Autodesk Fusion 360 part; units mm, degrees
(part 5 of 25)
  line L540 (19.5072, 53.213) -> (18.3388, 53.213)
  arc A1749 (22.1742, 53.7803) -> (22.1742, 53.8311) centre (22.1742, 53.8057) ccw
  arc A1750 (14.1676, 51.9684) -> (14.1676, 52.0192) centre (14.1676, 51.9938) ccw
  line L541 (22.1742, 53.6758) -> (22.1742, 53.9355)
  arc A1751 (18.3388, 53.8875) -> (18.3388, 53.8367) centre (18.3388, 53.8621) ccw
  arc A1752 (14.4272, 54.983) -> (14.4272, 55.0338) centre (14.4272, 55.0084) ccw
  arc A1753 (13.2334, 52.2534) -> (13.2842, 52.2534) centre (13.2588, 52.2534) ccw
  arc A1754 (19.5326, 54.7567) -> (19.4818, 54.7567) centre (19.5072, 54.7567) ccw
  arc A1755 (7.0605, 47.7158) -> (7.019, 47.6866) centre (7.0398, 47.7012) ccw
  arc A1756 (18.3388, 53.2384) -> (18.3388, 53.1876) centre (18.3388, 53.213) ccw
  arc A1757 (18.3265, 53.2352) -> (18.3511, 53.1908) centre (18.3388, 53.213) ccw
  arc A1758 (19.4818, 54.7567) -> (19.5326, 54.7567) centre (19.5072, 54.7567) ccw
  arc A1759 (18.3134, 54.7567) -> (18.3642, 54.7567) centre (18.3388, 54.7567) ccw
  arc A1760 (13.2588, 55.0338) -> (13.2588, 54.983) centre (13.2588, 55.0084) ccw
  line L542 (18.6634, 55.0813) -> (19.1826, 55.0813)
  arc A1761 (14.4526, 52.5131) -> (14.4018, 52.5131) centre (14.4272, 52.5131) ccw
  arc A1762 (13.2457, 53.0208) -> (13.2719, 52.9772) centre (13.2588, 52.999) ccw
  arc A1763 (19.5072, 53.1876) -> (19.5072, 53.2384) centre (19.5072, 53.213) ccw
  arc A1764 (7.4038, 46.5328) -> (7.4546, 46.5328) centre (7.4292, 46.5328) ccw
  arc A1765 (18.3642, 54.7567) -> (18.3134, 54.7567) centre (18.3388, 54.7567) ccw
  arc A1766 (18.3134, 54.4322) -> (18.3642, 54.4322) centre (18.3388, 54.4322) ccw
  arc A1767 (18.6634, 55.1067) -> (18.6634, 55.0559) centre (18.6634, 55.0813) ccw
  arc A1768 (18.6634, 55.0813) -> (18.3388, 54.7567) centre (18.6634, 54.7567) ccw
  line L543 (21.0058, 54.4336) -> (22.1742, 55.0827)
  arc A1769 (11.8618, 52.2534) -> (11.9126, 52.2534) centre (11.8872, 52.2534) ccw
  arc A1770 (19.5072, 53.8367) -> (19.5072, 53.8875) centre (19.5072, 53.8621) ccw
  line L544 (14.1676, 51.9938) -> (13.5184, 51.9938)
  arc A1771 (6.3103, 47.6932) -> (6.2621, 47.7092) centre (6.2862, 47.7012) ccw
  arc A1772 (13.2842, 52.5131) -> (13.2334, 52.5131) centre (13.2588, 52.5131) ccw
  arc A1773 (13.2588, 53.8033) -> (13.2588, 53.7525) centre (13.2588, 53.7779) ccw
  line L545 (18.3388, 53.213) -> (19.5072, 53.8621)
  arc A1774 (13.5184, 52.0192) -> (13.5184, 51.9684) centre (13.5184, 51.9938) ccw
  line L546 (11.8872, 52.5131) -> (11.8872, 52.2534)
  arc A1775 (19.5072, 54.4068) -> (19.5072, 54.4576) centre (19.5072, 54.4322) ccw
  arc A1776 (14.4018, 52.2534) -> (14.4526, 52.2534) centre (14.4272, 52.2534) ccw
  arc A1777 (14.1676, 51.9938) -> (14.4272, 52.2534) centre (14.1676, 52.2534) ccw
  line L547 (13.2588, 52.999) -> (13.9079, 53.3885)
  arc A1778 (14.4272, 54.3339) -> (14.4272, 54.3847) centre (14.4272, 54.3593) ccw
  line L548 (19.5072, 53.8621) -> (18.3388, 53.8621)
  arc A1779 (22.1822, 52.8672) -> (22.1662, 52.9154) centre (22.1742, 52.8913) ccw
  line L549 (19.5072, 54.7567) -> (19.5072, 54.4322)
  arc A1780 (22.1662, 52.8672) -> (22.1822, 52.9154) centre (22.1742, 52.8913) ccw
  arc A1781 (18.3388, 52.2534) -> (18.5984, 51.9938) centre (18.5984, 52.2534) ccw
  line L550 (14.4272, 52.999) -> (13.2588, 52.999)
  arc A1782 (13.921, 53.3667) -> (13.8948, 53.4103) centre (13.9079, 53.3885) ccw
  arc A1783 (19.5195, 53.8399) -> (19.4949, 53.8843) centre (19.5072, 53.8621) ccw
  arc A1784 (19.5072, 54.7567) -> (19.1826, 55.0813) centre (19.1826, 54.7567) ccw
  arc A1785 (19.1826, 55.1067) -> (19.1826, 55.0559) centre (19.1826, 55.0813) ccw
  arc A1786 (13.2588, 53.0244) -> (13.2588, 52.9736) centre (13.2588, 52.999) ccw
  line L551 (13.2588, 53.7779) -> (14.4272, 53.7779)
  arc A1787 (14.4272, 53.7525) -> (14.4272, 53.8033) centre (14.4272, 53.7779) ccw
  arc A1788 (18.6634, 55.0559) -> (18.6634, 55.1067) centre (18.6634, 55.0813) ccw
  line L552 (18.3388, 54.4322) -> (18.3388, 54.7567)
  arc A1789 (18.3388, 54.4576) -> (18.3388, 54.4068) centre (18.3388, 54.4322) ccw
  arc A1790 (6.6516, 46.5248) -> (6.6998, 46.5408) centre (6.6757, 46.5328) ccw
  arc A1791 (19.4818, 54.4322) -> (19.5326, 54.4322) centre (19.5072, 54.4322) ccw
  arc A1792 (19.1826, 55.0559) -> (19.1826, 55.1067) centre (19.1826, 55.0813) ccw
  arc A1793 (14.4526, 52.2534) -> (14.4018, 52.2534) centre (14.4272, 52.2534) ccw
  arc A1794 (13.5184, 51.9684) -> (13.5184, 52.0192) centre (13.5184, 51.9938) ccw
  line L553 (13.2588, 52.2534) -> (13.2588, 52.5131)
  arc A1795 (13.2588, 52.2534) -> (13.5184, 51.9938) centre (13.5184, 52.2534) ccw
  arc A1796 (13.2842, 52.2534) -> (13.2334, 52.2534) centre (13.2588, 52.2534) ccw
  line L554 (13.9079, 53.3885) -> (13.2588, 53.7779)
  line L555 (14.4272, 52.5131) -> (14.4272, 52.2534)
  arc A1797 (13.2719, 53.7997) -> (13.2457, 53.7562) centre (13.2588, 53.7779) ccw
  arc A1798 (13.8948, 53.3667) -> (13.921, 53.4103) centre (13.9079, 53.3885) ccw
  line L556 (14.4272, 54.3593) -> (13.2588, 54.3593)
  line L557 (13.2588, 54.3593) -> (14.4272, 55.0084)
  arc A1799 (16.9926, 53.5987) -> (16.9418, 53.5987) centre (16.9672, 53.5987) ccw
  arc A1800 (16.7076, 51.9938) -> (16.9672, 52.2534) centre (16.7076, 52.2534) ccw
  line L558 (16.9672, 52.9496) -> (16.9672, 53.5987)
  arc A1801 (11.9126, 52.2534) -> (11.8618, 52.2534) centre (11.8872, 52.2534) ccw
  arc A1802 (15.8242, 52.2534) -> (15.7734, 52.2534) centre (15.7988, 52.2534) ccw
  arc A1803 (14.1676, 52.0192) -> (14.1676, 51.9684) centre (14.1676, 51.9938) ccw
  line L559 (11.8872, 52.9496) -> (11.8872, 53.5987)
  arc A1804 (10.6934, 52.2534) -> (10.7442, 52.2534) centre (10.7188, 52.2534) ccw
  arc A1805 (63.6552, 12.3105) -> (63.6044, 12.3105) centre (63.6298, 12.3105) ccw
  arc A1806 (16.9672, 53.2488) -> (16.9672, 53.2996) centre (16.9672, 53.2742) ccw
  arc A1807 (11.8707, 52.9303) -> (11.9037, 52.969) centre (11.8872, 52.9497) ccw
  line L560 (15.7988, 52.2534) -> (15.7988, 52.5131)
  line L561 (16.9672, 52.5131) -> (16.9672, 52.2534)
  line L562 (16.0584, 52.9496) -> (15.7988, 53.2742)
  arc A1808 (10.7188, 52.2534) -> (10.9784, 51.9938) centre (10.9784, 52.2534) ccw
  arc A1809 (10.9706, 52.9255) -> (10.9863, 52.9738) centre (10.9784, 52.9497) ccw
  line L563 (11.2381, 53.5014) -> (11.8872, 52.9496)
  arc A1810 (14.4272, 52.9736) -> (14.4272, 53.0244) centre (14.4272, 52.999) ccw
  line L564 (14.4272, 55.0084) -> (13.2588, 55.0084)
  arc A1811 (13.2588, 54.3847) -> (13.2588, 54.3339) centre (13.2588, 54.3593) ccw
  arc A1812 (16.9418, 52.9496) -> (16.9926, 52.9496) centre (16.9672, 52.9496) ccw
  arc A1813 (10.7442, 52.5131) -> (10.6934, 52.5131) centre (10.7188, 52.5131) ccw
  arc A1814 (16.9926, 52.2534) -> (16.9418, 52.2534) centre (16.9672, 52.2534) ccw
  arc A1815 (11.0109, 53.5733) -> (11.0109, 53.6241) centre (11.0109, 53.5987) ccw
  line L565 (15.7988, 53.2742) -> (16.9672, 53.2742)
  arc A1816 (13.2465, 54.3815) -> (13.2711, 54.3371) centre (13.2588, 54.3593) ccw
  arc A1817 (14.4395, 54.9862) -> (14.4149, 55.0306) centre (14.4272, 55.0084) ccw
  arc A1818 (10.7442, 53.3066) -> (10.6934, 53.3066) centre (10.7188, 53.3066) ccw
  arc A1819 (63.6044, 10.2362) -> (63.6552, 10.2362) centre (63.6298, 10.2362) ccw
  arc A1820 (63.6552, 9.7197) -> (63.6044, 9.7197) centre (63.6298, 9.7197) ccw
  arc A1821 (11.9126, 53.5987) -> (11.8618, 53.5987) centre (11.8872, 53.5987) ccw
  arc A1822 (11.6276, 51.9684) -> (11.6276, 52.0192) centre (11.6276, 51.9938) ccw
  arc A1823 (10.9784, 52.0192) -> (10.9784, 51.9684) centre (10.9784, 51.9938) ccw
  arc A1824 (11.2545, 53.5207) -> (11.2216, 53.482) centre (11.2381, 53.5014) ccw
  arc A1825 (16.0584, 52.0192) -> (16.0584, 51.9684) centre (16.0584, 51.9938) ccw
  arc A1826 (63.6552, 11.0151) -> (63.6044, 11.0151) centre (63.6298, 11.0151) ccw
  arc A1827 (16.7076, 52.0192) -> (16.7076, 51.9684) centre (16.7076, 51.9938) ccw
  arc A1828 (10.6934, 53.3066) -> (10.7442, 53.3066) centre (10.7188, 53.3066) ccw
  arc A1829 (15.7988, 52.2534) -> (16.0584, 51.9938) centre (16.0584, 52.2534) ccw
  arc A1830 (16.0386, 52.9338) -> (16.0783, 52.9655) centre (16.0585, 52.9497) ccw
  arc A1831 (16.9418, 52.2534) -> (16.9926, 52.2534) centre (16.9672, 52.2534) ccw
  line L566 (16.7076, 51.9938) -> (16.0584, 51.9938)
  line L567 (63.6298, 10.2362) -> (63.6298, 11.0151)
  arc A1832 (11.0109, 53.6241) -> (11.0109, 53.5733) centre (11.0109, 53.5987) ccw
  line L568 (19.5072, 54.4322) -> (18.3388, 54.4322)
  arc A1833 (15.8242, 52.5131) -> (15.7734, 52.5131) centre (15.7988, 52.5131) ccw
  arc A1834 (11.2197, 53.4838) -> (11.2565, 53.5189) centre (11.2381, 53.5014) ccw
  arc A1835 (15.7988, 53.2996) -> (15.7988, 53.2488) centre (15.7988, 53.2742) ccw
  arc A1836 (10.7188, 53.3066) -> (10.9784, 52.9496) centre (11.094, 53.3066) ccw
  arc A1837 (16.0584, 51.9684) -> (16.0584, 52.0192) centre (16.0584, 51.9938) ccw
  arc A1838 (16.7076, 51.9684) -> (16.7076, 52.0192) centre (16.7076, 51.9938) ccw
  line L569 (63.6298, 8.9408) -> (63.6298, 9.7197)
  arc A1839 (10.7442, 52.2534) -> (10.6934, 52.2534) centre (10.7188, 52.2534) ccw
  line L570 (11.6276, 51.9938) -> (10.9784, 51.9938)
  arc A1840 (15.7734, 52.2534) -> (15.8242, 52.2534) centre (15.7988, 52.2534) ccw
  arc A1841 (11.6276, 51.9938) -> (11.8872, 52.2534) centre (11.6276, 52.2534) ccw
  line L571 (63.6298, 11.5316) -> (63.6298, 12.3105)
  arc A1842 (11.0109, 53.5987) -> (10.7188, 53.3066) centre (11.0109, 53.3066) ccw
  arc A1843 (11.8618, 52.9496) -> (11.9126, 52.9496) centre (11.8872, 52.9496) ccw
  arc A1844 (63.6044, 11.5316) -> (63.6552, 11.5316) centre (63.6298, 11.5316) ccw
  arc A1845 (63.6044, 8.9408) -> (63.6552, 8.9408) centre (63.6298, 8.9408) ccw
  line L572 (63.6298, 12.827) -> (63.6298, 13.6059)
  line L573 (68.7098, 8.9408) -> (68.7098, 9.7197)
  arc A1846 (15.8186, 53.29) -> (15.779, 53.2583) centre (15.7988, 53.2742) ccw
  arc A1847 (45.9813, 26.1699) -> (46.0259, 26.1456) centre (46.0036, 26.1577) ccw
  line L574 (45.5168, 27.1408) -> (45.5168, 27.66)
  line L575 (68.7098, 12.827) -> (68.7098, 13.6059)
  arc A1848 (10.9784, 51.9684) -> (10.9784, 52.0192) centre (10.9784, 51.9938) ccw
  line L576 (66.1698, 12.827) -> (66.1698, 13.6059)
  arc A1849 (11.2381, 53.5014) -> (11.0109, 53.5987) centre (11.011, 53.285) ccw
  arc A1850 (45.5422, 26.2876) -> (45.4914, 26.2876) centre (45.5168, 26.2876) ccw
  arc A1851 (45.5168, 27.1662) -> (45.5168, 27.1154) centre (45.5168, 27.1408) ccw
  arc A1852 (46.6852, 27.1154) -> (46.6852, 27.1662) centre (46.6852, 27.1408) ccw
  arc A1853 (46.5229, 25.9955) -> (46.6852, 26.385) centre (46.1367, 26.385) ccw
  arc A1854 (46.505, 26.0135) -> (46.5408, 25.9775) centre (46.5229, 25.9955) ccw
  arc A1855 (46.6598, 26.385) -> (46.7106, 26.385) centre (46.6852, 26.385) ccw
  arc A1856 (46.1765, 26.5277) -> (46.2203, 26.5019) centre (46.1984, 26.5148) ccw
  line L577 (10.7188, 52.2534) -> (10.7188, 52.5131)
  arc A1857 (66.1952, 12.3105) -> (66.1444, 12.3105) centre (66.1698, 12.3105) ccw
  arc A1858 (66.1952, 9.7197) -> (66.1444, 9.7197) centre (66.1698, 9.7197) ccw
  arc A1859 (66.1952, 13.6059) -> (66.1444, 13.6059) centre (66.1698, 13.6059) ccw
  arc A1860 (46.4256, 26.6192) -> (46.4256, 26.67) centre (46.4256, 26.6446) ccw
  line L578 (68.7098, 11.5316) -> (68.7098, 12.3105)
  arc A1861 (68.6844, 11.5316) -> (68.7352, 11.5316) centre (68.7098, 11.5316) ccw
  arc A1862 (45.7764, 26.028) -> (46.0036, 26.1578) centre (45.7764, 26.2917) ccw
  arc A1863 (45.6345, 26.5645) -> (45.5938, 26.5949) centre (45.6142, 26.5797) ccw
  arc A1864 (68.6844, 10.2362) -> (68.7352, 10.2362) centre (68.7098, 10.2362) ccw
  line L579 (63.6298, 14.1224) -> (63.6298, 14.9013)
  line L580 (68.7098, 10.2362) -> (68.7098, 11.0151)
  arc A1865 (66.1952, 11.0151) -> (66.1444, 11.0151) centre (66.1698, 11.0151) ccw
  arc A1866 (68.7352, 13.6059) -> (68.6844, 13.6059) centre (68.7098, 13.6059) ccw
  arc A1867 (66.1444, 14.1224) -> (66.1952, 14.1224) centre (66.1698, 14.1224) ccw
  arc A1868 (68.6844, 12.827) -> (68.7352, 12.827) centre (68.7098, 12.827) ccw
  arc A1869 (68.7352, 9.7197) -> (68.6844, 9.7197) centre (68.7098, 9.7197) ccw
  arc A1870 (63.6044, 14.1224) -> (63.6552, 14.1224) centre (63.6298, 14.1224) ccw
  line L581 (66.1698, 10.2362) -> (66.1698, 11.0151)
  arc A1871 (45.5422, 27.66) -> (45.4914, 27.66) centre (45.5168, 27.66) ccw
  line L582 (46.1984, 26.5148) -> (46.0036, 26.1578)
  arc A1872 (66.1444, 11.5316) -> (66.1952, 11.5316) centre (66.1698, 11.5316) ccw
  arc A1873 (46.7106, 26.385) -> (46.6598, 26.385) centre (46.6852, 26.385) ccw
  line L583 (66.1698, 11.5316) -> (66.1698, 12.3105)
  arc A1874 (46.6852, 26.385) -> (46.4256, 26.6446) centre (46.4256, 26.385) ccw
  arc A1875 (68.7352, 11.0151) -> (68.6844, 11.0151) centre (68.7098, 11.0151) ccw
  arc A1876 (68.7352, 12.3105) -> (68.6844, 12.3105) centre (68.7098, 12.3105) ccw
  line L584 (66.1698, 8.9408) -> (66.1698, 9.7197)
  arc A1877 (68.7352, 14.9013) -> (68.6844, 14.9013) centre (68.7098, 14.9013) ccw
  arc A1878 (45.6142, 26.5797) -> (45.5168, 26.2876) centre (46.0036, 26.2876) ccw
  arc A1879 (66.1952, 14.9013) -> (66.1444, 14.9013) centre (66.1698, 14.9013) ccw
  arc A1880 (45.7764, 26.0533) -> (45.7764, 26.0026) centre (45.7764, 26.028) ccw
  arc A1881 (63.6552, 13.6059) -> (63.6044, 13.6059) centre (63.6298, 13.6059) ccw
  arc A1882 (16.9926, 52.5131) -> (16.9418, 52.5131) centre (16.9672, 52.5131) ccw
  arc A1883 (11.9126, 52.5131) -> (11.8618, 52.5131) centre (11.8872, 52.5131) ccw
  arc A1884 (63.6552, 14.9013) -> (63.6044, 14.9013) centre (63.6298, 14.9013) ccw
  line L585 (46.6852, 27.1408) -> (45.5168, 27.1408)
  line L586 (68.7098, 14.1224) -> (68.7098, 14.9013)
  arc A1885 (46.7106, 27.66) -> (46.6598, 27.66) centre (46.6852, 27.66) ccw
  arc A1886 (45.4914, 26.2876) -> (45.5422, 26.2876) centre (45.5168, 26.2876) ccw
  arc A1887 (66.1444, 10.2362) -> (66.1952, 10.2362) centre (66.1698, 10.2362) ccw
  arc A1888 (11.6276, 52.0192) -> (11.6276, 51.9684) centre (11.6276, 51.9938) ccw
  arc A1889 (46.4256, 26.67) -> (46.4256, 26.6192) centre (46.4256, 26.6446) ccw
  arc A1890 (45.4914, 27.1408) -> (45.5422, 27.1408) centre (45.5168, 27.1408) ccw
  arc A1891 (63.6044, 12.827) -> (63.6552, 12.827) centre (63.6298, 12.827) ccw
  line L587 (46.0361, 27.1408) -> (46.0361, 27.5302)
  line L588 (66.1698, 14.1224) -> (66.1698, 14.9013)
  arc A1892 (66.1444, 12.827) -> (66.1952, 12.827) centre (66.1698, 12.827) ccw
  arc A1893 (46.2207, 26.5026) -> (46.1761, 26.5269) centre (46.1984, 26.5148) ccw
  line L589 (46.6852, 27.66) -> (46.6852, 27.1408)
  line L590 (48.5902, 28.091) -> (47.4218, 28.091)
  arc A1894 (45.8414, 30.4405) -> (45.8414, 30.3897) centre (45.8414, 30.4151) ccw
  arc A1895 (47.4416, 29.6125) -> (47.402, 29.5808) centre (47.4218, 29.5966) ccw
  arc A1896 (46.0107, 27.1408) -> (46.0615, 27.1408) centre (46.0361, 27.1408) ccw
  arc A1897 (45.4914, 28.461) -> (45.5422, 28.461) centre (45.5168, 28.461) ccw
  arc A1898 (45.8414, 31.0896) -> (45.8414, 31.0388) centre (45.8414, 31.0642) ccw
  arc A1899 (47.4472, 28.4155) -> (47.3964, 28.4155) centre (47.4218, 28.4155) ccw
  arc A1900 (46.3606, 30.3897) -> (46.3606, 30.4405) centre (46.3606, 30.4151) ccw
  line L591 (47.7464, 28.7401) -> (48.2656, 28.7401)
  arc A1901 (47.4218, 29.622) -> (47.4218, 29.5712) centre (47.4218, 29.5966) ccw
  line L592 (48.5902, 29.2721) -> (48.5902, 29.9212)
  arc A1902 (45.5168, 28.1619) -> (45.5168, 28.1111) centre (45.5168, 28.1365) ccw
  arc A1903 (66.1444, 8.9408) -> (66.1952, 8.9408) centre (66.1698, 8.9408) ccw
  arc A1904 (45.5168, 26.2876) -> (45.7764, 26.028) centre (45.7764, 26.2876) ccw
  arc A1905 (46.3606, 30.4405) -> (46.3606, 30.3897) centre (46.3606, 30.4151) ccw
  line L593 (46.6852, 29.5966) -> (45.5168, 29.9861)
  arc A1906 (47.3964, 28.4155) -> (47.4472, 28.4155) centre (47.4218, 28.4155) ccw
  line L594 (48.5902, 28.4155) -> (48.5902, 28.091)
  arc A1907 (45.4914, 28.1365) -> (45.5422, 28.1365) centre (45.5168, 28.1365) ccw
  arc A1908 (46.0255, 26.1449) -> (45.9818, 26.1707) centre (46.0037, 26.1578) ccw
  arc A1909 (48.5648, 28.4156) -> (48.6156, 28.4155) centre (48.5902, 28.4155) ccw
  line L595 (46.6852, 28.1365) -> (45.5168, 28.1365)
  arc A1910 (47.7464, 28.7147) -> (47.7464, 28.7655) centre (47.7464, 28.7401) ccw
  line L596 (45.5168, 29.2072) -> (46.6852, 29.5966)
  arc A1911 (45.5248, 30.0102) -> (45.5088, 29.962) centre (45.5168, 29.9861) ccw
  arc A1912 (46.4256, 26.6446) -> (46.1984, 26.5148) centre (46.4256, 26.3809) ccw
  arc A1913 (47.7464, 28.7401) -> (47.4218, 28.4155) centre (47.7464, 28.4155) ccw
  arc A1914 (48.5902, 28.0656) -> (48.5902, 28.1164) centre (48.5902, 28.091) ccw
  arc A1915 (46.6932, 29.5726) -> (46.6772, 29.6207) centre (46.6852, 29.5967) ccw
  arc A1916 (46.1405, 28.1365) -> (46.1913, 28.1365) centre (46.1659, 28.1365) ccw
  arc A1917 (46.6598, 27.1408) -> (46.7106, 27.1408) centre (46.6852, 27.1408) ccw
  arc A1918 (46.6852, 28.1111) -> (46.6852, 28.1619) centre (46.6852, 28.1365) ccw
  line L597 (47.4218, 28.091) -> (47.4218, 28.4155)
  arc A1919 (45.5088, 29.2313) -> (45.5248, 29.1831) centre (45.5168, 29.2072) ccw
  arc A1920 (46.3606, 30.4151) -> (46.3606, 31.0642) centre (46.3606, 30.7396) ccw
  arc A1921 (48.2656, 28.7147) -> (48.2656, 28.7655) centre (48.2656, 28.7401) ccw
  line L598 (46.1659, 28.461) -> (46.1659, 28.1365)
  line L599 (45.5168, 28.1365) -> (45.5168, 28.461)
  arc A1922 (48.2656, 28.7655) -> (48.2656, 28.7147) centre (48.2656, 28.7401) ccw
  line L600 (45.8414, 31.0642) -> (46.3606, 31.0642)
  arc A1923 (48.5902, 28.4155) -> (48.2656, 28.7401) centre (48.2656, 28.4155) ccw
  arc A1924 (47.6616, 29.2562) -> (47.7013, 29.288) centre (47.6814, 29.2721) ccw
  line L601 (47.4218, 29.5966) -> (48.5902, 29.5966)
  arc A1925 (45.5422, 28.461) -> (45.4914, 28.461) centre (45.5168, 28.461) ccw
  arc A1926 (45.8414, 31.0642) -> (45.8414, 30.4151) centre (45.8414, 30.7396) ccw
  arc A1927 (68.6844, 14.1224) -> (68.7352, 14.1224) centre (68.7098, 14.1224) ccw
  arc A1928 (47.3964, 28.091) -> (47.4472, 28.091) centre (47.4218, 28.091) ccw
  arc A1929 (48.5648, 28.091) -> (48.6156, 28.091) centre (48.5902, 28.091) ccw
  arc A1930 (45.7764, 26.0025) -> (45.7764, 26.0534) centre (45.7764, 26.028) ccw
  line L602 (47.6814, 29.2721) -> (47.4218, 29.5966)
  arc A1931 (46.1659, 28.461) -> (45.5168, 28.461) centre (45.8414, 28.461) ccw
  arc A1932 (46.3606, 31.0896) -> (46.3606, 31.0388) centre (46.3606, 31.0642) ccw
  arc A1933 (45.8414, 30.3897) -> (45.8414, 30.4405) centre (45.8414, 30.4151) ccw
  arc A1934 (68.6844, 8.9408) -> (68.7352, 8.9408) centre (68.7098, 8.9408) ccw
  arc A1935 (48.5902, 29.5712) -> (48.5902, 29.622) centre (48.5902, 29.5966) ccw
  arc A1936 (46.6772, 29.5726) -> (46.6932, 29.6207) centre (46.6852, 29.5966) ccw
  arc A1937 (47.7464, 28.7655) -> (47.7464, 28.7147) centre (47.7464, 28.7401) ccw
  arc A1938 (46.0615, 27.5302) -> (46.0107, 27.5302) centre (46.0361, 27.5302) ccw
  arc A1939 (48.6156, 28.4155) -> (48.5648, 28.4155) centre (48.5902, 28.4155) ccw
  line L603 (46.6852, 28.7856) -> (46.1659, 28.5259)
  arc A1940 (46.3606, 31.0388) -> (46.3606, 31.0896) centre (46.3606, 31.0642) ccw
  arc A1941 (46.1913, 28.461) -> (46.1405, 28.461) centre (46.1659, 28.461) ccw
  arc A1942 (46.6966, 28.7628) -> (46.6738, 28.8083) centre (46.6852, 28.7856) ccw
  line L604 (46.3606, 30.4151) -> (45.8414, 30.4151)
  arc A1943 (46.1546, 28.5486) -> (46.1773, 28.5032) centre (46.166, 28.5259) ccw
  arc A1944 (54.2535, 39.2374) -> (54.2028, 39.2374) centre (54.2282, 39.2374) ccw
  arc A1945 (48.5902, 30.7142) -> (48.5902, 30.765) centre (48.5902, 30.7396) ccw
  arc A1946 (55.0198, 38.8874) -> (55.0198, 38.9382) centre (55.0198, 38.9128) ccw
  line L605 (57.3142, 38.9128) -> (57.3142, 40.0812)
  arc A1947 (47.4218, 30.765) -> (47.4218, 30.7142) centre (47.4218, 30.7396) ccw
  arc A1948 (53.5536, 39.2374) -> (53.6044, 39.2374) centre (53.579, 39.2374) ccw
  line L606 (55.4092, 38.9128) -> (55.0198, 38.9128)
  arc A1949 (48.6156, 29.9212) -> (48.5648, 29.9212) centre (48.5902, 29.9212) ccw
  line L607 (47.6814, 30.4151) -> (47.4218, 30.7396)
  line L608 (53.579, 39.2374) -> (53.579, 39.7566)
  arc A1950 (53.579, 39.2374) -> (54.2281, 39.2374) centre (53.9036, 39.2374) ccw
  line L609 (55.9074, 38.9128) -> (56.167, 38.9128)
  line L610 (55.9074, 40.0812) -> (56.167, 40.0812)
  arc A1951 (56.167, 40.0558) -> (56.167, 40.1066) centre (56.167, 40.0812) ccw
  arc A1952 (55.9074, 38.9382) -> (55.9074, 38.8874) centre (55.9074, 38.9128) ccw
  line L611 (52.6288, 40.0812) -> (52.6288, 38.9128)
  arc A1953 (57.292, 38.9005) -> (57.3364, 38.9251) centre (57.3142, 38.9128) ccw
  line L612 (55.0198, 40.0812) -> (55.4092, 40.0812)
  arc A1954 (53.6044, 39.7566) -> (53.5536, 39.7566) centre (53.579, 39.7566) ccw
  arc A1955 (54.2027, 39.7566) -> (54.2535, 39.7566) centre (54.2281, 39.7566) ccw
  line L613 (55.4092, 39.5619) -> (55.4092, 38.9128)
  arc A1956 (55.0198, 38.9382) -> (55.0198, 38.8874) centre (55.0198, 38.9128) ccw
  arc A1957 (56.0626, 40.0812) -> (56.0118, 40.0812) centre (56.0372, 40.0812) ccw
  arc A1958 (45.8414, 31.0388) -> (45.8414, 31.0896) centre (45.8414, 31.0642) ccw
  line L614 (56.6651, 38.9128) -> (56.6651, 40.0812)
  arc A1959 (53.1481, 38.8874) -> (53.1481, 38.9382) centre (53.1481, 38.9128) ccw
  line L615 (47.4218, 30.7396) -> (48.5902, 30.7396)
  arc A1960 (54.2028, 39.2374) -> (54.2535, 39.2374) centre (54.2282, 39.2374) ccw
  arc A1961 (54.7855, 39.8216) -> (54.7347, 39.8216) centre (54.7601, 39.8216) ccw
  arc A1962 (54.7347, 39.8216) -> (54.7855, 39.8216) centre (54.7601, 39.8216) ccw
  arc A1963 (47.4416, 30.7555) -> (47.402, 30.7238) centre (47.4218, 30.7396) ccw
  arc A1964 (56.0118, 38.9128) -> (56.0626, 38.9128) centre (56.0372, 38.9128) ccw
  line L616 (54.2281, 39.7566) -> (54.2281, 39.2374)
  arc A1965 (47.6616, 30.3992) -> (47.7013, 30.431) centre (47.6814, 30.4151) ccw
  arc A1966 (52.6288, 38.9382) -> (52.6288, 38.8874) centre (52.6288, 38.9128) ccw
  arc A1967 (55.3838, 38.9128) -> (55.4346, 38.9128) centre (55.4092, 38.9128) ccw
  line L617 (54.7601, 39.1724) -> (54.7601, 39.8216)
  arc A1968 (55.0198, 40.0558) -> (55.0198, 40.1066) centre (55.0198, 40.0812) ccw
  arc A1969 (53.5536, 39.7566) -> (53.6044, 39.7566) centre (53.579, 39.7566) ccw
  arc A1970 (55.4092, 40.0558) -> (55.4092, 40.1066) centre (55.4092, 40.0812) ccw
  arc A1971 (55.0198, 40.0812) -> (54.7601, 39.8216) centre (55.0198, 39.8215) ccw
  arc A1972 (48.5648, 30.4151) -> (48.6156, 30.4151) centre (48.5902, 30.4151) ccw
  arc A1973 (48.6156, 31.0642) -> (48.5648, 31.0642) centre (48.5902, 31.0642) ccw
  arc A1974 (55.4092, 38.8874) -> (55.4092, 38.9382) centre (55.4092, 38.9128) ccw
  arc A1975 (54.7347, 39.1724) -> (54.7855, 39.1724) centre (54.7601, 39.1724) ccw
  arc A1976 (54.7855, 39.1724) -> (54.7347, 39.1724) centre (54.7601, 39.1724) ccw
  line L618 (56.0372, 40.0812) -> (56.0372, 38.9128)
  arc A1977 (56.6905, 40.0812) -> (56.6397, 40.0812) centre (56.6651, 40.0812) ccw
  arc A1978 (46.1405, 28.461) -> (46.1913, 28.461) centre (46.1659, 28.461) ccw
  arc A1979 (55.0198, 40.1066) -> (55.0198, 40.0558) centre (55.0198, 40.0812) ccw
  arc A1980 (48.5648, 29.2721) -> (48.6156, 29.2721) centre (48.5902, 29.2721) ccw
  arc A1981 (54.2535, 39.7566) -> (54.2028, 39.7566) centre (54.2282, 39.7566) ccw
  line L619 (48.5902, 30.4151) -> (48.5902, 31.0642)
  arc A1982 (47.4218, 28.1164) -> (47.4218, 28.0656) centre (47.4218, 28.091) ccw
  line L620 (55.2145, 39.5619) -> (55.4092, 39.5619)
  arc A1983 (55.4092, 39.5365) -> (55.4092, 39.5873) centre (55.4092, 39.5619) ccw
  arc A1984 (56.6873, 40.0935) -> (56.6429, 40.0689) centre (56.6651, 40.0812) ccw
  line L621 (56.6651, 40.0812) -> (57.3142, 38.9128)
  arc A1985 (54.7601, 39.1724) -> (55.0198, 38.9128) centre (55.0198, 39.1725) ccw
  arc A1986 (52.6542, 40.0812) -> (52.6034, 40.0812) centre (52.6288, 40.0812) ccw
  arc A1987 (55.9074, 40.1066) -> (55.9074, 40.0558) centre (55.9074, 40.0812) ccw
  arc A1988 (56.6397, 38.9128) -> (56.6905, 38.9128) centre (56.6651, 38.9128) ccw
  arc A1989 (19.2984, 13.1318) -> (19.2984, 13.1826) centre (19.2984, 13.1572) ccw
  arc A1990 (57.2888, 38.9128) -> (57.3396, 38.9128) centre (57.3142, 38.9128) ccw
  arc A1991 (18.9992, 13.1572) -> (18.9484, 13.1572) centre (18.9738, 13.1572) ccw
  arc A1992 (57.8984, 39.0497) -> (57.8984, 39.1005) centre (57.8984, 39.0751) ccw
  arc A1993 (21.115, 11.9888) -> (21.1658, 11.9888) centre (21.1404, 11.9888) ccw
  arc A1994 (57.8589, 39.5944) -> (57.8081, 39.5944) centre (57.8335, 39.5944) ccw
  arc A1995 (21.6597, 12.6125) -> (21.6597, 12.6633) centre (21.6597, 12.6379) ccw
  line L622 (57.8335, 39.5944) -> (57.8984, 39.5944)
  arc A1996 (55.4346, 39.5619) -> (55.3838, 39.5619) centre (55.4092, 39.5619) ccw
  arc A1997 (18.9484, 11.9888) -> (18.9992, 11.9888) centre (18.9738, 11.9888) ccw
  arc A1998 (19.2984, 12.5335) -> (19.2984, 12.4827) centre (19.2984, 12.5081) ccw
  arc A1999 (57.8335, 39.5549) -> (57.8335, 39.5041) centre (57.8335, 39.5295) ccw
  arc A2000 (57.8984, 38.9848) -> (57.8984, 39.0356) centre (57.8984, 39.0102) ccw
  arc A2001 (57.873, 39.5295) -> (57.9238, 39.5295) centre (57.8984, 39.5295) ccw
  arc A2002 (20.1498, 12.0142) -> (20.1498, 11.9634) centre (20.1498, 11.9888) ccw
  line L623 (57.8335, 39.5295) -> (57.8335, 39.5944)
  arc A2003 (20.6691, 11.9634) -> (20.6691, 12.0142) centre (20.6691, 11.9888) ccw
  line L624 (57.8984, 39.5944) -> (57.8984, 39.5295)
  arc A2004 (57.8081, 39.5295) -> (57.8589, 39.5295) centre (57.8335, 39.5295) ccw
  line L625 (18.9738, 11.9888) -> (18.9738, 13.1572)
  line L626 (21.1404, 13.1572) -> (21.6597, 13.1572)
  arc A2005 (21.6597, 13.1318) -> (21.6597, 13.1826) centre (21.6597, 13.1572) ccw
  arc A2006 (20.6691, 13.1318) -> (20.6691, 13.1826) centre (20.6691, 13.1572) ccw
  arc A2007 (57.9238, 39.0751) -> (57.873, 39.0751) centre (57.8984, 39.0751) ccw
  arc A2008 (55.2145, 39.5873) -> (55.2145, 39.5365) centre (55.2145, 39.5619) ccw
  arc A2009 (57.8589, 39.0751) -> (57.8081, 39.0751) centre (57.8335, 39.0751) ccw
  arc A2010 (52.6034, 38.9128) -> (52.6542, 38.9128) centre (52.6288, 38.9128) ccw
  line L627 (57.8984, 39.5295) -> (57.8335, 39.5295)
  line L628 (57.8984, 39.0102) -> (57.8335, 39.0102)
  arc A2011 (18.9738, 13.1826) -> (18.9738, 13.1318) centre (18.9738, 13.1572) ccw
  arc A2012 (53.6044, 39.2374) -> (53.5536, 39.2374) centre (53.579, 39.2374) ccw
  arc A2013 (21.1658, 13.1572) -> (21.115, 13.1572) centre (21.1404, 13.1572) ccw
  line L629 (21.1404, 11.9888) -> (21.1404, 13.1572)
  line L630 (19.6229, 11.9888) -> (19.3633, 12.5081)
  arc A2014 (57.9238, 39.5944) -> (57.873, 39.5944) centre (57.8984, 39.5944) ccw
  arc A2015 (19.6002, 11.9774) -> (19.6456, 12.0002) centre (19.6229, 11.9888) ccw
  arc A2016 (20.1752, 13.1572) -> (20.1244, 13.1572) centre (20.1498, 13.1572) ccw
  arc A2017 (19.2984, 12.5081) -> (19.2984, 13.1572) centre (19.2984, 12.8327) ccw
  line L631 (20.1498, 11.9888) -> (20.1498, 13.1572)
  arc A2018 (57.3396, 40.0812) -> (57.2888, 40.0812) centre (57.3142, 40.0812) ccw
  arc A2019 (54.2281, 39.7566) -> (53.579, 39.7566) centre (53.9036, 39.7566) ccw
  line L632 (20.1498, 12.6379) -> (20.5393, 12.6379)
  line L633 (20.6691, 11.9888) -> (20.1498, 11.9888)
  line L634 (19.2984, 12.5081) -> (18.9738, 12.5081)
  arc A2020 (57.8081, 39.0102) -> (57.8589, 39.0102) centre (57.8335, 39.0102) ccw
  arc A2021 (57.8984, 39.569) -> (57.8984, 39.6198) centre (57.8984, 39.5944) ccw
  arc A2022 (20.5393, 12.6125) -> (20.5393, 12.6633) centre (20.5393, 12.6379) ccw
  arc A2023 (18.9738, 12.5335) -> (18.9738, 12.4827) centre (18.9738, 12.5081) ccw
  arc A2024 (19.2984, 12.4827) -> (19.2984, 12.5335) centre (19.2984, 12.5081) ccw
  line L635 (57.8335, 39.0751) -> (57.8984, 39.0751)
  line L636 (18.9738, 13.1572) -> (19.2984, 13.1572)
  arc A2025 (20.1244, 11.9888) -> (20.1752, 11.9888) centre (20.1498, 11.9888) ccw
  arc A2026 (56.167, 38.8874) -> (56.167, 38.9382) centre (56.167, 38.9128) ccw
  arc A2027 (20.1498, 13.1826) -> (20.1498, 13.1318) centre (20.1498, 13.1572) ccw
  arc A2028 (57.8335, 39.1005) -> (57.8335, 39.0497) centre (57.8335, 39.0751) ccw
  line L637 (20.1498, 13.1572) -> (20.6691, 13.1572)
  arc A2029 (57.8984, 39.5041) -> (57.8984, 39.5549) centre (57.8984, 39.5295) ccw
  arc A2030 (20.1498, 12.6633) -> (20.1498, 12.6125) centre (20.1498, 12.6379) ccw
  arc A2031 (21.1404, 13.1826) -> (21.1404, 13.1318) centre (21.1404, 13.1572) ccw
  line L638 (57.8335, 39.0102) -> (57.8335, 39.0751)
  arc A2032 (57.8335, 39.0356) -> (57.8335, 38.9848) centre (57.8335, 39.0102) ccw
  line L639 (52.6288, 38.9128) -> (53.1481, 38.9128)
  arc A2033 (19.386, 12.5194) -> (19.3405, 12.4967) centre (19.3633, 12.5081) ccw
  arc A2034 (57.873, 39.0102) -> (57.9238, 39.0102) centre (57.8984, 39.0102) ccw
  arc A2035 (25.3164, 13.1572) -> (25.2656, 13.1572) centre (25.291, 13.1572) ccw
  arc A2036 (26.7285, 13.1826) -> (26.7285, 13.1318) centre (26.7285, 13.1572) ccw
  arc A2037 (24.822, 11.9634) -> (24.822, 12.0142) centre (24.822, 11.9888) ccw
  arc A2038 (25.9179, 11.9765) -> (25.9623, 12.0011) centre (25.9401, 11.9888) ccw
  arc A2039 (24.3027, 13.1826) -> (24.3027, 13.1318) centre (24.3027, 13.1572) ccw
  arc A2040 (26.9881, 11.9634) -> (26.9881, 12.0142) centre (26.9881, 11.9888) ccw
  arc A2041 (23.4513, 13.1318) -> (23.4513, 13.1826) centre (23.4513, 13.1572) ccw
  line L640 (23.4513, 12.5081) -> (23.1267, 12.5081)
  arc A2042 (23.1521, 13.1572) -> (23.1013, 13.1572) centre (23.1267, 13.1572) ccw
  arc A2043 (25.2656, 11.9888) -> (25.3164, 11.9888) centre (25.291, 11.9888) ccw
  arc A2044 (26.4688, 12.2484) -> (26.7285, 11.9888) centre (26.7285, 12.2485) ccw
  arc A2045 (25.9147, 11.9888) -> (25.9655, 11.9888) centre (25.9401, 11.9888) ccw
  arc A2046 (21.1404, 12.6633) -> (21.1404, 12.6125) centre (21.1404, 12.6379) ccw
  line L641 (22.131, 13.1572) -> (22.6503, 13.1572)
  line L642 (25.291, 13.1572) -> (25.9401, 11.9888)
  arc A2047 (23.1267, 12.5335) -> (23.1267, 12.4827) centre (23.1267, 12.5081) ccw
  arc A2048 (22.131, 13.1826) -> (22.131, 13.1318) centre (22.131, 13.1572) ccw
  line L643 (23.1267, 13.1572) -> (23.4513, 13.1572)
  arc A2049 (23.4513, 12.5081) -> (23.4513, 13.1572) centre (23.4513, 12.8327) ccw
  arc A2050 (22.1564, 13.1572) -> (22.1056, 13.1572) centre (22.131, 13.1572) ccw
  arc A2051 (24.822, 13.1318) -> (24.822, 13.1826) centre (24.822, 13.1572) ccw
  arc A2052 (57.8335, 39.6198) -> (57.8335, 39.569) centre (57.8335, 39.5944) ccw
  arc A2053 (27.9843, 11.9634) -> (27.9843, 12.0142) centre (27.9843, 11.9888) ccw
  arc A2054 (25.9655, 13.1572) -> (25.9147, 13.1572) centre (25.9401, 13.1572) ccw
  arc A2055 (23.5389, 12.5194) -> (23.4934, 12.4967) centre (23.5162, 12.5081) ccw
  arc A2056 (23.4513, 12.4827) -> (23.4513, 12.5335) centre (23.4513, 12.5081) ccw
  arc A2057 (23.4513, 12.5335) -> (23.4513, 12.4827) centre (23.4513, 12.5081) ccw
  arc A2058 (26.7285, 13.1318) -> (26.7285, 13.1826) centre (26.7285, 13.1572) ccw
  arc A2059 (22.5205, 12.6125) -> (22.5205, 12.6633) centre (22.5205, 12.6379) ccw
  line L644 (24.3027, 12.6379) -> (24.6922, 12.6379)
  arc A2060 (24.3027, 12.0142) -> (24.3027, 11.9634) centre (24.3027, 11.9888) ccw
  arc A2061 (24.6922, 12.6125) -> (24.6922, 12.6633) centre (24.6922, 12.6379) ccw
  arc A2062 (22.6503, 13.1318) -> (22.6503, 13.1826) centre (22.6503, 13.1572) ccw
  line L645 (22.6503, 11.9888) -> (22.131, 11.9888)
  line L646 (23.7758, 11.9888) -> (23.5162, 12.5081)
  arc A2063 (27.465, 12.0142) -> (27.465, 11.9634) centre (27.465, 11.9888) ccw
  line L647 (23.1267, 11.9888) -> (23.1267, 13.1572)
  line L648 (27.465, 11.9888) -> (27.465, 13.1572)
  line L649 (21.1404, 12.6379) -> (21.6597, 12.6379)
  arc A2064 (26.7285, 11.9634) -> (26.7285, 12.0142) centre (26.7285, 11.9888) ccw
  line L650 (22.131, 12.6379) -> (22.5205, 12.6379)
  arc A2065 (26.4942, 12.2484) -> (26.4434, 12.2484) centre (26.4688, 12.2484) ccw
  arc A2066 (27.4904, 13.1572) -> (27.4396, 13.1572) centre (27.465, 13.1572) ccw
  arc A2067 (26.7285, 12.0142) -> (26.7285, 11.9634) centre (26.7285, 11.9888) ccw
  line L651 (24.3027, 11.9888) -> (24.3027, 13.1572)
  line L652 (22.131, 11.9888) -> (22.131, 13.1572)
  arc A2068 (23.1013, 11.9888) -> (23.1521, 11.9888) centre (23.1267, 11.9888) ccw
  arc A2069 (24.3027, 12.6633) -> (24.3027, 12.6125) centre (24.3027, 12.6379) ccw
  arc A2070 (22.131, 12.6633) -> (22.131, 12.6125) centre (22.131, 12.6379) ccw
  arc A2071 (23.1267, 13.1826) -> (23.1267, 13.1318) centre (23.1267, 13.1572) ccw
  arc A2072 (22.131, 12.0142) -> (22.131, 11.9634) centre (22.131, 11.9888) ccw
  line L653 (57.8984, 39.0751) -> (57.8984, 39.0102)
  line L654 (24.822, 11.9888) -> (24.3027, 11.9888)
  arc A2073 (23.4513, 13.1826) -> (23.4513, 13.1318) centre (23.4513, 13.1572) ccw
  arc A2074 (22.6503, 11.9634) -> (22.6503, 12.0142) centre (22.6503, 11.9888) ccw
  arc A2075 (24.3281, 13.1572) -> (24.2773, 13.1572) centre (24.3027, 13.1572) ccw
  line L655 (27.9843, 11.9888) -> (27.465, 11.9888)
  arc A2076 (25.3132, 13.1695) -> (25.2688, 13.1449) centre (25.291, 13.1572) ccw
  line L656 (26.9881, 11.9888) -> (26.7285, 11.9888)
  arc A2077 (19.2984, 13.1826) -> (19.2984, 13.1318) centre (19.2984, 13.1572) ccw
  arc A2078 (22.1056, 11.9888) -> (22.1564, 11.9888) centre (22.131, 11.9888) ccw
  arc A2079 (23.7531, 11.9774) -> (23.7985, 12.0002) centre (23.7758, 11.9888) ccw
  line L657 (25.291, 11.9888) -> (25.291, 13.1572)
  arc A2080 (24.2773, 11.9888) -> (24.3281, 11.9888) centre (24.3027, 11.9888) ccw
  line L658 (24.3027, 13.1572) -> (24.822, 13.1572)
  arc A2081 (19.2984, 10.5777) -> (19.2984, 10.6285) centre (19.2984, 10.6031) ccw
  arc A2082 (21.3939, 10.0584) -> (21.3939, 10.1092) centre (21.3939, 10.0838) ccw
  arc A2083 (20.0838, 10.3434) -> (20.033, 10.3434) centre (20.0584, 10.3434) ccw
  arc A2084 (21.0693, 11.2776) -> (21.0693, 11.2268) centre (21.0693, 11.2522) ccw
  line L659 (26.4688, 12.2484) -> (26.4688, 12.8976)
  arc A2085 (27.4396, 11.9888) -> (27.4904, 11.9888) centre (27.465, 11.9888) ccw
  arc A2086 (19.2984, 10.6031) -> (19.2984, 11.2522) centre (19.2984, 10.9277) ccw
  line L660 (21.0693, 10.0838) -> (21.0693, 11.2522)
  arc A2087 (21.0439, 10.0838) -> (21.0947, 10.0838) centre (21.0693, 10.0838) ccw
  line L661 (27.465, 12.6379) -> (27.8545, 12.6379)
  arc A2088 (26.4942, 12.8976) -> (26.4434, 12.8976) centre (26.4688, 12.8976) ccw
  arc A2089 (19.2984, 10.6285) -> (19.2984, 10.5777) centre (19.2984, 10.6031) ccw
  arc A2090 (27.465, 13.1826) -> (27.465, 13.1318) centre (27.465, 13.1572) ccw
  line L662 (21.0693, 10.7329) -> (21.3939, 10.7329)
  arc A2091 (20.0838, 10.9926) -> (20.033, 10.9926) centre (20.0584, 10.9926) ccw
  arc A2092 (21.3939, 11.2268) -> (21.3939, 11.2776) centre (21.3939, 11.2522) ccw
  arc A2093 (21.3939, 11.2776) -> (21.3939, 11.2268) centre (21.3939, 11.2522) ccw
  arc A2094 (21.3939, 10.1092) -> (21.3939, 10.0584) centre (21.3939, 10.0838) ccw
  arc A2095 (21.3939, 10.7583) -> (21.3939, 10.7075) centre (21.3939, 10.7329) ccw
  arc A2096 (26.4434, 12.2484) -> (26.4942, 12.2484) centre (26.4688, 12.2484) ccw
  arc A2097 (18.9738, 10.6285) -> (18.9738, 10.5777) centre (18.9738, 10.6031) ccw
  arc A2098 (20.3181, 11.2268) -> (20.3181, 11.2776) centre (20.3181, 11.2522) ccw
  arc A2099 (21.3939, 10.7075) -> (21.3939, 10.7583) centre (21.3939, 10.7329) ccw
  arc A2100 (20.3181, 11.2522) -> (20.0584, 10.9926) centre (20.3181, 10.9925) ccw
  arc A2101 (26.7285, 13.1572) -> (26.4688, 12.8976) centre (26.7285, 12.8975) ccw
  arc A2102 (27.465, 12.6633) -> (27.465, 12.6125) centre (27.465, 12.6379) ccw
  line L663 (21.0693, 11.2522) -> (21.3939, 11.2522)
  arc A2103 (21.0693, 10.7583) -> (21.0693, 10.7075) centre (21.0693, 10.7329) ccw
  arc A2104 (20.5777, 11.2268) -> (20.5777, 11.2776) centre (20.5777, 11.2522) ccw
  arc A2105 (19.2984, 11.2268) -> (19.2984, 11.2776) centre (19.2984, 11.2522) ccw
  line L664 (20.5777, 10.0838) -> (20.3181, 10.0838)
  arc A2106 (20.033, 10.9926) -> (20.0838, 10.9926) centre (20.0584, 10.9926) ccw
  arc A2107 (26.4434, 12.8976) -> (26.4942, 12.8976) centre (26.4688, 12.8976) ccw
  arc A2108 (20.3181, 10.1092) -> (20.3181, 10.0584) centre (20.3181, 10.0838) ccw
  arc A2109 (20.3181, 10.0584) -> (20.3181, 10.1092) centre (20.3181, 10.0838) ccw
  arc A2110 (20.5777, 10.0584) -> (20.5777, 10.1092) centre (20.5777, 10.0838) ccw
  arc A2111 (21.0947, 11.2522) -> (21.0439, 11.2522) centre (21.0693, 11.2522) ccw
  line L665 (19.2984, 10.6031) -> (18.9738, 10.6031)
  arc A2112 (26.9881, 13.1318) -> (26.9881, 13.1826) centre (26.9881, 13.1572) ccw
  line L666 (27.465, 13.1572) -> (27.9843, 13.1572)
  arc A2113 (21.0693, 10.1092) -> (21.0693, 10.0584) centre (21.0693, 10.0838) ccw
  arc A2114 (21.3939, 10.7583) -> (21.3939, 10.7075) centre (21.3939, 10.7329) ccw
  line L667 (20.0584, 10.3434) -> (20.0584, 10.9926)
  arc A2115 (20.0584, 10.3434) -> (20.3181, 10.0838) centre (20.3181, 10.3435) ccw
  arc A2116 (21.3939, 10.0838) -> (21.3939, 10.7329) centre (21.3939, 10.4084) ccw
  line L668 (21.3939, 10.0838) -> (21.0693, 10.0838)
  line L669 (26.7285, 13.1572) -> (26.9881, 13.1572)
  line L670 (18.9738, 11.2522) -> (19.2984, 11.2522)
  line L671 (25.9401, 11.9888) -> (25.9401, 13.1572)
  arc A2117 (20.3181, 11.2776) -> (20.3181, 11.2268) centre (20.3181, 11.2522) ccw
  arc A2118 (18.9992, 11.2522) -> (18.9484, 11.2522) centre (18.9738, 11.2522) ccw
  arc A2119 (18.9484, 10.0838) -> (18.9992, 10.0838) centre (18.9738, 10.0838) ccw
  line L672 (18.9738, 10.0838) -> (18.9738, 11.2522)
  arc A2120 (20.033, 10.3434) -> (20.0838, 10.3434) centre (20.0584, 10.3434) ccw
  arc A2121 (19.2984, 11.2776) -> (19.2984, 11.2268) centre (19.2984, 11.2522) ccw
  line L673 (20.3181, 11.2522) -> (20.5777, 11.2522)
  arc A2122 (18.9738, 11.2776) -> (18.9738, 11.2268) centre (18.9738, 11.2522) ccw
  arc A2123 (22.6314, 42.8554) -> (22.6822, 42.8554) centre (22.6568, 42.8554) ccw
  arc A2124 (21.3939, 10.7329) -> (21.3939, 11.2522) centre (21.3939, 10.9926) ccw
  arc A2125 (27.8545, 12.6125) -> (27.8545, 12.6633) centre (27.8545, 12.6379) ccw
  arc A2126 (27.9843, 13.1318) -> (27.9843, 13.1826) centre (27.9843, 13.1572) ccw
  arc A2127 (23.1761, 42.5704) -> (23.1761, 42.6212) centre (23.1761, 42.5958) ccw
  arc A2128 (22.9164, 43.7388) -> (22.9164, 43.7896) centre (22.9164, 43.7642) ccw
  arc A2129 (22.9814, 41.1988) -> (22.9814, 41.2496) centre (22.9814, 41.2242) ccw
  arc A2130 (22.6568, 41.2496) -> (22.6568, 41.1988) centre (22.6568, 41.2242) ccw
  arc A2131 (22.6568, 37.5412) -> (22.6568, 37.4904) centre (22.6568, 37.5158) ccw
  arc A2132 (22.6568, 40.0812) -> (22.6568, 40.0304) centre (22.6568, 40.0558) ccw
  arc A2133 (22.9814, 40.7303) -> (22.9814, 40.6795) centre (22.9814, 40.7049) ccw
  arc A2134 (22.6822, 43.5046) -> (22.6314, 43.5046) centre (22.6568, 43.5046) ccw
  line L674 (22.9164, 43.7642) -> (23.1761, 43.7642)
  arc A2135 (23.1761, 37.4904) -> (23.1761, 37.5412) centre (23.1761, 37.5158) ccw
  arc A2136 (22.6568, 38.1903) -> (22.6568, 38.1395) centre (22.6568, 38.1649) ccw
  arc A2137 (22.6822, 42.8554) -> (22.6314, 42.8554) centre (22.6568, 42.8554) ccw
  line L675 (22.6568, 37.5158) -> (22.6568, 38.6842)
  arc A2138 (72.1043, 51.3715) -> (72.0408, 51.3715) centre (72.0726, 51.3715) ccw
  arc A2139 (23.1761, 38.6588) -> (23.1761, 38.7096) centre (23.1761, 38.6842) ccw
  arc A2140 (72.3265, 52.2287) -> (72.3265, 52.2923) centre (72.3265, 52.2605) ccw
  line L676 (72.5805, 51.1175) -> (72.3265, 51.1175)
  arc A2141 (72.3265, 52.2605) -> (72.0725, 52.0065) centre (72.3265, 52.0065) ccw
  arc A2142 (73.0287, 51.1493) -> (73.0287, 51.0857) centre (73.0287, 51.1175) ccw
  line L677 (72.0725, 51.3715) -> (72.0725, 52.0065)
  arc A2143 (22.6314, 37.5158) -> (22.6822, 37.5158) centre (22.6568, 37.5158) ccw
  arc A2144 (72.0408, 52.0065) -> (72.1043, 52.0065) centre (72.0726, 52.0065) ccw
  arc A2145 (72.5805, 52.2287) -> (72.5805, 52.2923) centre (72.5805, 52.2605) ccw
  arc A2146 (73.6637, 51.0857) -> (73.6637, 51.1493) centre (73.6637, 51.1175) ccw
  arc A2147 (73.3145, 51.1175) -> (73.378, 51.1175) centre (73.3462, 51.1175) ccw
  arc A2148 (73.378, 52.2605) -> (73.3145, 52.2605) centre (73.3462, 52.2605) ccw
  arc A2149 (22.9164, 42.5704) -> (22.9164, 42.6212) centre (22.9164, 42.5958) ccw
  line L678 (22.6568, 40.7049) -> (22.9814, 40.7049)
  arc A2150 (22.9814, 40.0558) -> (22.9814, 40.7049) centre (22.9814, 40.3803) ccw
  line L679 (22.6568, 40.0558) -> (22.6568, 41.2242)
  line L680 (22.6568, 38.6842) -> (23.1761, 38.6842)
  arc A2151 (22.6822, 38.6842) -> (22.6314, 38.6842) centre (22.6568, 38.6842) ccw
  arc A2152 (72.1043, 52.0065) -> (72.0408, 52.0065) centre (72.0726, 52.0065) ccw
  arc A2153 (22.9814, 41.2496) -> (22.9814, 41.1988) centre (22.9814, 41.2242) ccw
  arc A2154 (22.9814, 40.7049) -> (22.9814, 41.2242) centre (22.9814, 40.9646) ccw
  arc A2155 (72.3265, 52.2923) -> (72.3265, 52.2287) centre (72.3265, 52.2605) ccw
  line L681 (22.6568, 38.1649) -> (23.0463, 38.1649)
  line L682 (73.0287, 52.0065) -> (73.3462, 52.2605)
  line L683 (23.1761, 42.5958) -> (22.9164, 42.5958)
  arc A2156 (22.9164, 42.6212) -> (22.9164, 42.5704) centre (22.9164, 42.5958) ccw
  arc A2157 (22.6314, 40.0558) -> (22.6822, 40.0558) centre (22.6568, 40.0558) ccw
  arc A2158 (22.6314, 43.5046) -> (22.6822, 43.5046) centre (22.6568, 43.5046) ccw
  arc A2159 (72.3265, 51.1493) -> (72.3265, 51.0857) centre (72.3265, 51.1175) ccw
  arc A2160 (72.5805, 51.0857) -> (72.5805, 51.1493) centre (72.5805, 51.1175) ccw
  line L684 (22.6568, 42.8554) -> (22.6568, 43.5046)
  arc A2161 (22.6568, 42.8554) -> (22.9164, 42.5958) centre (22.9164, 42.8554) ccw
  arc A2162 (22.9164, 43.7896) -> (22.9164, 43.7388) centre (22.9164, 43.7642) ccw
  arc A2163 (22.6568, 38.7096) -> (22.6568, 38.6588) centre (22.6568, 38.6842) ccw
  arc A2164 (22.6822, 41.2242) -> (22.6314, 41.2242) centre (22.6568, 41.2242) ccw
  line L685 (73.3462, 52.2605) -> (73.3462, 51.1175)
  arc A2165 (23.0463, 38.1395) -> (23.0463, 38.1903) centre (23.0463, 38.1649) ccw
  arc A2166 (72.0725, 51.3715) -> (72.3265, 51.1175) centre (72.3265, 51.3715) ccw
  arc A2167 (22.9814, 40.0812) -> (22.9814, 40.0304) centre (22.9814, 40.0558) ccw
  line L686 (22.9814, 40.0558) -> (22.6568, 40.0558)
  arc A2168 (22.9814, 40.7303) -> (22.9814, 40.6795) centre (22.9814, 40.7049) ccw
  line L687 (23.1761, 37.5158) -> (22.6568, 37.5158)
  arc A2169 (22.9164, 43.7642) -> (22.6568, 43.5046) centre (22.9164, 43.5046) ccw
  arc A2170 (23.1761, 43.7388) -> (23.1761, 43.7896) centre (23.1761, 43.7642) ccw
  arc A2171 (22.6568, 40.7303) -> (22.6568, 40.6795) centre (22.6568, 40.7049) ccw
  arc A2172 (22.9814, 40.0304) -> (22.9814, 40.0812) centre (22.9814, 40.0558) ccw
  line L688 (22.6568, 41.2242) -> (22.9814, 41.2242)
  arc A2173 (72.0408, 51.3715) -> (72.1043, 51.3715) centre (72.0726, 51.3715) ccw
  arc A2174 (22.9814, 40.6795) -> (22.9814, 40.7303) centre (22.9814, 40.7049) ccw
  arc A2175 (73.3661, 52.2357) -> (73.3264, 52.2853) centre (73.3463, 52.2605) ccw
  arc A2176 (73.0089, 52.0313) -> (73.0486, 51.9817) centre (73.0288, 52.0065) ccw
  line L689 (72.3265, 52.2605) -> (72.5805, 52.2605)
  arc A2177 (55.0545, 20.5422) -> (55.0545, 20.4788) centre (55.0545, 20.5105) ccw
  arc A2178 (56.106, 20.5105) -> (55.7567, 20.2565) centre (56.106, 20.1434) ccw
  arc A2179 (11.9697, 38.608) -> (12.0333, 38.608) centre (12.0015, 38.608) ccw
  arc A2180 (11.176, 38.9255) -> (10.8585, 38.608) centre (11.176, 38.608) ccw
  arc A2181 (11.9697, 38.2905) -> (12.0333, 38.2905) centre (12.0015, 38.2905) ccw
  arc A2182 (56.3917, 19.3358) -> (56.3917, 19.3992) centre (56.3917, 19.3675) ccw
  line L690 (12.0015, 38.2905) -> (10.8585, 38.2905)
  arc A2183 (11.1443, 40.0748) -> (11.1443, 40.1384) centre (11.1443, 40.1066) ccw
  arc A2184 (11.3871, 40.0355) -> (11.3459, 39.9872) centre (11.3665, 40.0114) ccw
  arc A2185 (12.0015, 38.608) -> (11.684, 38.9255) centre (11.684, 38.608) ccw
  arc A2186 (11.176, 38.8937) -> (11.176, 38.9573) centre (11.176, 38.9255) ccw
  arc A2187 (11.684, 38.9573) -> (11.684, 38.8937) centre (11.684, 38.9255) ccw
  line L691 (56.2965, 20.0025) -> (55.7567, 19.3675)
  arc A2188 (56.36, 20.2248) -> (56.4235, 20.2248) centre (56.3918, 20.2248) ccw
  arc A2189 (55.0545, 19.3358) -> (55.0545, 19.3992) centre (55.0545, 19.3675) ccw
  arc A2190 (55.3085, 19.3358) -> (55.3085, 19.3992) centre (55.3085, 19.3675) ccw
  arc A2191 (55.0545, 20.5105) -> (54.8005, 20.2565) centre (55.0545, 20.2565) ccw
  arc A2192 (55.7325, 19.3881) -> (55.7809, 19.3469) centre (55.7567, 19.3675) ccw
  arc A2193 (54.8323, 19.6215) -> (54.7687, 19.6215) centre (54.8005, 19.6215) ccw
  arc A2194 (56.106, 20.5422) -> (56.106, 20.4788) centre (56.106, 20.5105) ccw
  arc A2195 (55.0545, 19.3992) -> (55.0545, 19.3358) centre (55.0545, 19.3675) ccw
  arc A2196 (56.2746, 20.0255) -> (56.3184, 19.9795) centre (56.2965, 20.0025) ccw
  arc A2197 (56.4235, 20.2248) -> (56.36, 20.2247) centre (56.3918, 20.2248) ccw
  line L692 (54.8005, 19.6215) -> (54.8005, 20.2565)
  arc A2198 (54.7687, 19.6215) -> (54.8323, 19.6215) centre (54.8005, 19.6215) ccw
  arc A2199 (12.0015, 38.2587) -> (12.0015, 38.3223) centre (12.0015, 38.2905) ccw
  arc A2200 (55.0545, 20.4788) -> (55.0545, 20.5422) centre (55.0545, 20.5105) ccw
  arc A2201 (10.8585, 38.3223) -> (10.8585, 38.2587) centre (10.8585, 38.2905) ccw
  arc A2202 (11.176, 38.9573) -> (11.176, 38.8937) centre (11.176, 38.9255) ccw
  arc A2203 (11.1442, 40.1383) -> (11.1443, 40.0749) centre (11.1442, 40.1066) ccw
  arc A2204 (11.3665, 40.0114) -> (11.1443, 40.1066) centre (11.1444, 39.7998) ccw
  line L693 (55.0545, 20.5105) -> (55.3085, 20.5105)
  arc A2205 (54.7687, 20.2565) -> (54.8323, 20.2565) centre (54.8005, 20.2565) ccw
  arc A2206 (72.3265, 51.0857) -> (72.3265, 51.1493) centre (72.3265, 51.1175) ccw
  arc A2207 (56.2965, 20.0025) -> (56.3917, 20.2248) centre (56.0848, 20.2247) ccw
  arc A2208 (54.8005, 19.6215) -> (55.0545, 19.3675) centre (55.0545, 19.6215) ccw
  arc A2209 (55.7567, 19.3992) -> (55.7567, 19.3358) centre (55.7567, 19.3675) ccw
  arc A2210 (56.3207, 19.9819) -> (56.2723, 20.0231) centre (56.2965, 20.0025) ccw
  line L694 (12.0015, 39.4716) -> (12.0015, 40.1066)
  line L695 (10.8585, 38.2905) -> (10.8585, 38.608)
  arc A2211 (12.0333, 40.1066) -> (11.9697, 40.1066) centre (12.0015, 40.1066) ccw
  arc A2212 (10.8268, 39.8209) -> (10.8903, 39.8209) centre (10.8586, 39.8209) ccw
  arc A2213 (55.3085, 20.4788) -> (55.3085, 20.5422) centre (55.3085, 20.5105) ccw
  arc A2214 (10.8268, 38.608) -> (10.8903, 38.608) centre (10.8586, 38.608) ccw
  line L696 (55.7567, 19.3675) -> (56.3917, 19.3675)
  arc A2215 (11.1443, 40.1066) -> (10.8585, 39.8209) centre (11.1443, 39.8208) ccw
  arc A2216 (56.3917, 20.2248) -> (56.106, 20.5105) centre (56.106, 20.2248) ccw
  arc A2217 (43.9774, 31.3303) -> (44.017, 31.2807) centre (43.9972, 31.3055) ccw
  arc A2218 (10.8903, 38.608) -> (10.8268, 38.608) centre (10.8586, 38.608) ccw
  arc A2219 (56.106, 20.4788) -> (56.106, 20.5422) centre (56.106, 20.5105) ccw
  arc A2220 (11.684, 38.8937) -> (11.684, 38.9573) centre (11.684, 38.9255) ccw
  arc A2221 (12.0333, 38.608) -> (11.9697, 38.608) centre (12.0015, 38.608) ccw
  line L697 (55.3085, 19.3675) -> (55.0545, 19.3675)
  arc A2222 (11.3435, 39.9895) -> (11.3895, 40.0332) centre (11.3665, 40.0114) ccw
  arc A2223 (54.8323, 20.2565) -> (54.7687, 20.2565) centre (54.8005, 20.2565) ccw
  line L698 (11.176, 38.9255) -> (11.684, 38.9255)
  line L699 (73.0287, 51.1175) -> (73.6637, 51.1175)
  arc A2224 (11.9697, 39.4716) -> (12.0333, 39.4716) centre (12.0015, 39.4716) ccw
  line L700 (11.3665, 40.0114) -> (12.0015, 39.4716)
  arc A2225 (11.1027, 39.4414) -> (11.1223, 39.5018) centre (11.1125, 39.4716) ccw
  arc A2226 (10.8903, 39.8208) -> (10.8268, 39.8209) centre (10.8586, 39.8209) ccw
  arc A2227 (10.8268, 38.2905) -> (10.8903, 38.2905) centre (10.8586, 38.2905) ccw
  arc A2228 (55.7265, 20.2663) -> (55.7869, 20.2467) centre (55.7567, 20.2565) ccw
  line L701 (12.0015, 38.608) -> (12.0015, 38.2905)
  line L702 (71.2799, 44.5135) -> (71.2799, 44.0055)
  line L703 (42.3545, 30.4165) -> (42.1005, 30.9245)
  arc A2229 (42.037, 31.5278) -> (42.037, 31.5912) centre (42.037, 31.5595) ccw
  line L704 (42.037, 30.9245) -> (41.7195, 30.9245)
  arc A2230 (24.2264, 26.0668) -> (24.2264, 26.1303) centre (24.2264, 26.0985) ccw
  arc A2231 (41.7195, 30.9563) -> (41.7195, 30.8928) centre (41.7195, 30.9246) ccw
  arc A2232 (23.0505, 24.9555) -> (23.3045, 25.2095) centre (23.0505, 25.2095) ccw
  arc A2233 (23.0505, 24.9238) -> (23.0505, 24.9872) centre (23.0505, 24.9555) ccw
  arc A2234 (23.9724, 25.6223) -> (23.9724, 25.5588) centre (23.9724, 25.5906) ccw
  arc A2235 (43.4892, 30.3848) -> (43.4892, 30.4483) centre (43.4892, 30.4166) ccw
  line L705 (23.8454, 26.0985) -> (24.2264, 26.0985)
  arc A2236 (24.1629, 25.6223) -> (24.1629, 25.5588) centre (24.1629, 25.5906) ccw
  arc A2237 (41.7513, 31.5595) -> (41.6878, 31.5595) centre (41.7196, 31.5595) ccw
  arc A2238 (22.9235, 24.9872) -> (22.9235, 24.9238) centre (22.9235, 24.9555) ccw
  arc A2239 (24.1629, 24.9872) -> (24.1629, 24.9238) centre (24.1629, 24.9555) ccw
  arc A2240 (71.1199, 45.1398) -> (71.0588, 45.1572) centre (71.0894, 45.1485) ccw
  arc A2241 (24.2264, 25.5588) -> (24.2264, 25.6223) centre (24.2264, 25.5906) ccw
  line L706 (70.2945, 45.1485) -> (70.2945, 44.2595)
  line L707 (41.7195, 30.4165) -> (41.7195, 31.5595)
  arc A2242 (70.3263, 45.1485) -> (70.2627, 45.1485) centre (70.2945, 45.1485) ccw
  arc A2243 (70.3263, 44.2595) -> (70.2627, 44.2595) centre (70.2945, 44.2595) ccw
  line L708 (23.0505, 24.9555) -> (22.9235, 24.9555)
  line L709 (70.2945, 32.4485) -> (70.2945, 31.5595)
  line L710 (71.0894, 45.1485) -> (70.8354, 44.2595)